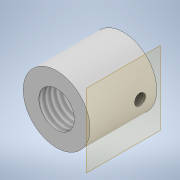
# Autodesk Inventor part: Glasdeckel
Saved by Autodesk Inventor 2021.3 (Build 253353000, 353)
## iProperties
Created: 2021-10-18
Part Number: Glasdeckel
Material: Generisch
Document SubType Name: Modeling
Designer: bhelg
Density: 1 g/cm^3
Appearance: Vorgabe
Author: bhelg
Autodesk Inventor part; units mm, degrees
note: some values were not read from the file. Chosen so that the rebuilt part matches the saved one: direction of "Bohrung1".
ref_plane "XZ Plane" through (0, 0, 0) normal (0, 1, 0) x (-1, 0, 0)
ref_plane "XY Plane" through (0, 0, 0) normal (0, 0, 1) x (1, 0, 0)
sketch "Skizze1" plane through (0, 0, 0) normal (0, 1, 0) x (-1, 0, 0)
  line L0 (4, 0) -> (4, -7.5)
  line L1 (4, -7.5) -> (3, -7.5)
  line L2 (7.5, -15) -> (7.5, 0)
  line L3 (7.5, 0) -> (4, 0)
  line L4 (0, 3.7992) -> (0, -25.1489)
  line L5 (7.5, -15) -> (3, -15)
  line L6 (3, -15) -> (3, -10)
  line L7 (3, -10) -> (3, -10)
  line L8 (3, -10) -> (3, -7.5)
  point P0 (0, 0)
  dimension "d6" = 4
  dimension "d9" = 4.5
  dimension "d10" = 5
  dimension "d15" = 6
  dimension "d16" = 15
  dimension "d17" = 7.5
  dimension "d18" = 15
  constraints: 18 end point, 5 perpendicular, 2 point on line, 1 horizontal, 1 parallel, 1 vertical
  measures "d6" distance from line of L0 point (0, 0)
  measures "d9" distance of L2.start L5.end
  measures "d10" distance of L5.end L6.end
  measures "d15" diameter of L8 L4
  measures "d16" diameter of L2 L4
  measures "d17" vertical distance of point (0, 0) L0.end
  measures "d18" distance between parallel lines of L3 L5
revolve "Umdrehung1" add sketch "Skizze1" angle 360 about axis through (0, 0, 3.7992) along (0, 0, -1)
thread "Gewinde1" size "M6x1" class "6H" standard "ANSI Metric M Profile" full length
thread "Gewinde2" size "M8x1.25" class "6H" standard "ANSI Metric M Profile" full length
ref_plane "Arbeitsebene1" through (7.5, 0, 0) normal (1, 0, 0) x (0, 1, 0)
sketch "Skizze3" plane through (7.5, 0, 0) normal (1, 0, 0) x (0, 1, 0)
  line L0 (-4, -7.5) -> (4, -7.5) projected
  line L1 (-7.5, -15) -> (7.5, -15) projected
  line L2 (0, 0) -> (0, -15)
  line L3 (-3, -15) -> (3, -15) projected
  point P0 (0, -11.25)
  dimension "d20" = 3.75
  constraints: 2 end point, 1 midpoint, 1 point on line
  measures "d20" distance from line of L1 point (0, -11.25)
hole "Bohrung1" at (7.5, 0, -11.25) direction (-1, 0, 0) diameter 2.459 end up to surface thread size "M3x0.5" class "6H" standard "ISO Metric profile"
